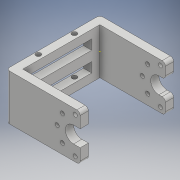
# Autodesk Inventor part: elbow_gear
Saved by Autodesk Inventor 2018 (Build 220112000, 112)
## iProperties
Created: 2020-09-07
Part Number: elbow_gear
Material: 일반
Document SubType Name: Modeling
Designer: j3jjj
Density: 1 g/cm^3
Appearance: 기본값
Author: j3jjj
Autodesk Inventor part; units mm, degrees
ref_plane "YZ Plane" through (0, 0, 0) normal (1, 0, 0) x (0, 1, 0)
ref_plane "XZ Plane" through (0, 0, 0) normal (0, 1, 0) x (-1, 0, 0)
ref_plane "XY Plane" through (0, 0, 0) normal (0, 0, 1) x (1, 0, 0)
sketch "스케치1" plane through (0, 0, 0) normal (0, 1, 0) x (-1, 0, 0)
  line L0 (22.5, -14) -> (-22.5, -14)
  line L1 (-22.5, -14) -> (-22.5, 14)
  line L2 (-22.5, 14) -> (22.5, 14)
  line L3 (22.5, 14) -> (22.5, -14)
  point P0 (0, 0)
  dimension "d0" = 28
  dimension "d1" = 45
  dimension "d2" = 14
  dimension "d3" = 22.5
  constraints: 8 end point, 2 parallel, 1 horizontal, 1 perpendicular
  measures "d0" distance between parallel lines of L0 L2
  measures "d1" distance between parallel lines of L1 L3
  measures "d2" distance from line of L2 point (0, 0)
  measures "d3" distance from line of point (0, 0) L3
extrude "돌출1" add sketch "스케치1" along normal blind 5
sketch "스케치2" plane through (0, 5, 0) normal (0, 1, 0) x (1, 0, 0)
  circle A0 centre (18.5, 0) radius 5
  line L0 (18.5, 5) -> (22.5, 5)
  line L1 (22.5, 5) -> (22.5, -5)
  line L2 (22.5, -5) -> (18.5, -5)
  line L3 (18.5, -5) -> (18.5, 5)
  line L4 (22.5, -14) -> (22.5, 14) projected
  point P0 (0, 0)
  dimension "d6" = 10
  dimension "d7" = 0
  dimension "d8" = 10
  dimension "d9" = 5
  dimension "d10" = 4
  dimension "d11" = 0
  constraints: 8 end point, 2 parallel, 1 centre point, 1 horizontal, 1 perpendicular
  measures "d6" diameter of A0
  measures "d7" distance between parallel lines of L1 L4
  measures "d8" distance between parallel lines of L0 L2
  measures "d9" distance from line of point (0, 0) L2
  measures "d10" distance between parallel lines of L1 L3
  measures "d11" distance from line of A0.centre L3
extrude "돌출2" cut sketch "스케치2" against normal blind 100
sketch "스케치3" plane through (0, 5, 0) normal (0, 1, 0) x (1, 0, 0)
  circle A0 centre (19.5, 11) radius 1.25
  line L0 (22.5, 5) -> (22.5, 14) projected
  line L1 (22.5, 14) -> (-22.5, 14) projected
  line L2 (0, 0) -> (4.9885, 0)
  circle A1 centre (19.5, -11) radius 1.25
  circle A2 centre (8.5, 0) radius 1.25
  line L3 (-22.5, -14) -> (22.5, -14) projected
  circle A3 centre (11.722, -7.778) radius 1.25
  line L4 (22.5, -14) -> (22.5, -5) projected
  circle A4 centre (11.722, 7.778) radius 1.25
  dimension "d14" = 2.5
  dimension "d15" = 3
  dimension "d16" = 3
  dimension "d17" = 14
  dimension "d18" = 2.5
  dimension "d19" = 14
  dimension "d20" = 10.778
  dimension "d21" = 6.222
  dimension "d22" = 2.5
  constraints: 5 centre point, 2 end point, 2 symmetric about line, 1 horizontal, 2 other
  measures "d14" diameter of A0
  measures "d15" distance from line of L0 A0.centre
  measures "d16" distance from line of L1 A0.centre
  measures "d17" distance from line of L0 A2.centre
  measures "d18" diameter of A2
  measures "d19" distance from line of L3 A2.centre
  measures "d20" distance from line of L4 A3.centre
  measures "d21" distance from line of L3 A3.centre
  measures "d22" diameter of A3
extrude "돌출3" cut sketch "스케치3" against normal blind 5
fillet "모깎기1" radius 2 4 edges at (22.5, 2.5, -14) (22.5, 2.5, 14) (22.5, 2.5, -5) (22.5, 2.5, 5)
sketch "스케치4" plane through (0, 0, 0) normal (0, -1, 0) x (1, 0, 0)
  line L0 (-22.5, -14) -> (20.5, -14) projected
  line L1 (20.5, 14) -> (-22.5, 14) projected
  line L2 (-22.5, -14) -> (-17.5, -14)
  line L3 (-17.5, -14) -> (-17.5, 14)
  line L4 (-17.5, 14) -> (-22.5, 14)
  line L5 (-22.5, 14) -> (-22.5, -14)
  point P0 (0, 0)
  dimension "d26" = 5
  constraints: 8 end point, 2 parallel, 1 horizontal, 1 perpendicular, 1 point on line
  measures "d26" distance between parallel lines of L5 L3
extrude "돌출4" add sketch "스케치4" along normal blind 52
fillet "모깎기2" radius 2 1 edges at (-22.5, 5, 0)
sketch "스케치5" plane through (-17.5, 0, 14) normal (1, 0, 0) x (0, 0, -1)
  point P0 (14, 0)
sketch "스케치6" plane through (-17.5, 0, 14) normal (1, 0, 0) x (0, 0, -1)
  line L0 (28, 0) -> (28, -52) projected
  line L1 (0, 0) -> (0, -52) projected
  line L2 (28, -52) -> (0, -52)
  line L3 (0, -52) -> (0, -47)
  line L4 (0, -47) -> (28, -47)
  line L5 (28, -47) -> (28, -52)
  point P0 (14, 0)
  dimension "d30" = 5
  constraints: 8 end point, 2 parallel, 1 horizontal, 1 perpendicular, 1 point on line
  measures "d30" distance between parallel lines of L2 L4
extrude "돌출5" add sketch "스케치6" along normal blind 40
sketch "스케치7" plane through (0, 0, 0) normal (0, -1, 0) x (1, 0, 0)
  circle A0 centre (19.5, -11) radius 1.25 projected
  circle A1 centre (19.5, -11) radius 1.25
  circle A2 centre (11.722, -7.778) radius 1.25 projected
  circle A3 centre (11.722, -7.778) radius 1.25
  circle A4 centre (8.5, 0) radius 1.25 projected
  circle A5 centre (8.5, 0) radius 1.25
  circle A6 centre (11.722, 7.778) radius 1.25 projected
  circle A7 centre (11.722, 7.778) radius 1.25
  circle A8 centre (19.5, 11) radius 1.25 projected
  circle A9 centre (19.5, 11) radius 1.25
  arc A10 (18.5, 5) -> (18.5, -5) centre (18.5, 0) ccw projected
  circle A11 centre (18.5, 0) radius 5
  line L0 (18.5, -5) -> (29.1098, -5)
  line L1 (29.1098, -5) -> (29.1098, 5)
  line L2 (29.1098, 5) -> (18.5, 5)
  line L3 (18.5, 5) -> (18.5, -5)
  point P0 (0, 0)
  constraints: 8 end point, 6 centre point, 6 coincident, 2 parallel, 1 horizontal, 1 perpendicular
extrude "돌출6" cut sketch "스케치7" along normal blind 200
fillet "모깎기4" radius 2 2 edges at (22.5, -49.5, 14) (22.5, -49.5, -14)
fillet "모깎기5" radius 2 1 edges at (-22.5, -52, 0)
sketch "스케치10" plane through (20.5, 0, 14) normal (0, 0, 1) x (1, 0, 0)
  circle A0 centre (-41, -12.5) radius 1.5
  circle A1 centre (-41, -34.5) radius 1.5
  line L0 (-32.0554, -23.5) -> (-2.5003, -23.5)
  line L1 (-43, 3) -> (-43, -50) projected
  point P0 (-20.5, 0)
  dimension "d54" = 3
  dimension "d55" = 3
  dimension "d56" = 22
  dimension "d57" = 23.5
  dimension "d58" = 11
  dimension "d59" = 2
  dimension "d60" = 2
  constraints: 2 centre point, 2 end point, 1 horizontal
  measures "d54" diameter of A1
  measures "d55" diameter of A0
  measures "d56" distance of A0.centre A1.centre
  measures "d57" distance from line of point (-20.5, 0) L0
  measures "d58" distance from line of L0 A1.centre
  measures "d59" distance from line of A1.centre L1
  measures "d60" distance from line of A0.centre L1
extrude "돌출9" cut sketch "스케치10" against normal blind 80
sketch "스케치11" plane through (-17.5, 0, 14) normal (1, 0, 0) x (0, 0, -1)
  line L0 (5, -42) -> (23, -42)
  line L1 (23, -42) -> (23, -5)
  line L2 (23, -5) -> (5, -5)
  line L3 (5, -5) -> (5, -42)
  line L4 (0, 0) -> (0, -47) projected
  line L5 (28, 0) -> (28, -47) projected
  line L6 (19, 0) -> (9, 0) projected
  line L7 (9, -47) -> (19, -47) projected
  line L8 (11, -42) -> (17, -42)
  line L9 (17, -42) -> (17, -5)
  line L10 (17, -5) -> (11, -5)
  line L11 (11, -5) -> (11, -42)
  point P0 (14, 0)
  dimension "d63" = 5
  dimension "d64" = 5
  dimension "d65" = 5
  dimension "d66" = 5
  dimension "d67" = 6
  dimension "d68" = 6
  constraints: 16 end point, 4 parallel, 2 horizontal, 2 perpendicular, 2 point on line
  measures "d63" distance between parallel lines of L3 L4
  measures "d64" distance between parallel lines of L5 L1
  measures "d65" distance between parallel lines of L6 L2
  measures "d66" distance between parallel lines of L0 L7
  measures "d67" distance between parallel lines of L11 L3
  measures "d68" distance between parallel lines of L1 L9
extrude "돌출10" cut sketch "스케치11" against normal blind 80 contours L3 L2 L11 L0 | L9 L2 L1 L0
sketch "스케치12" plane through (-17.5, -42, 3) normal (0, 0, 1) x (1, 0, 0)
  circle A0 centre (-3, 7.5) radius 1.5 projected
  circle A1 centre (-3, 7.5) radius 1.5
  circle A2 centre (-3, 29.5) radius 1.5 projected
  circle A3 centre (-3, 29.5) radius 1.5
  point P0 (17.5, 42)
  constraints: 2 centre point, 2 coincident
extrude "돌출11" add sketch "스케치12" against normal blind 6
